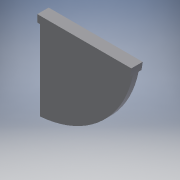
# Autodesk Inventor part: Control surface
Saved by Autodesk Inventor 2016 (Build 200138000, 138)
## iProperties
Created: 2015-09-03
Part Number: Control surface
Material: Generic
Document SubType Name: Modeling
Designer: Sudhar
Density: 1 g/cm^3
Appearance: Default
Author: Sudhar
Autodesk Inventor part; units mm, degrees
ref_plane "YZ Plane" through (0, 0, 0) normal (1, 0, 0) x (0, 1, 0)
ref_plane "XZ Plane" through (0, 0, 0) normal (0, 1, 0) x (-1, 0, 0)
ref_plane "XY Plane" through (0, 0, 0) normal (0, 0, 1) x (1, 0, 0)
sketch "Sketch1" plane through (0, 0, 0) normal (0, 0, 1) x (1, 0, 0)
  line L0 (12.2331, 11.5545) -> (-8.7602, 11.5545)
  line L1 (-8.7602, 11.5545) -> (-8.7602, -8.5579)
  arc A0 (-8.7602, -8.5579) -> (12.2331, 11.5545) centre (-10.663, 14.4408) ccw
  point P0 (0, 0)
  constraints: 4 end point, 2 point on circle, 1 centre point, 1 horizontal, 1 perpendicular
extrude "Extrusion1" add sketch "Sketch1" along normal mid plane 2.54
sketch "Sketch2" plane through (0, 0, 1.27) normal (0, 0, 1) x (1, 0, 0)
  line L0 (-8.7602, 11.5545) -> (-8.7602, -8.5579) projected
  line L1 (-8.7602, 9.9328) -> (11.9484, 9.8273)
  arc A0 (-8.7602, -8.5579) -> (12.2331, 11.5545) centre (-10.663, 14.4408) ccw projected
  point P0 (0, 0)
  constraints: 2 end point, 1 point on circle, 1 point on line
extrude "Extrusion2" cut sketch "Sketch2" against normal blind 0.635
sketch "Sketch3" plane through (0, 0, -1.27) normal (0, 0, -1) x (-1, 0, 0)
  line L0 (8.7602, 9.9328) -> (-11.9484, 9.8273) projected
  line L1 (8.7602, -8.5579) -> (8.7602, 11.5545) projected
  line L2 (8.7602, 9.9328) -> (8.7602, -8.5579)
  arc A0 (-11.9484, 9.8273) -> (8.7602, -8.5579) centre (10.663, 14.4408) ccw
  point P0 (0, 0)
  constraints: 2 end point, 2 point on circle, 1 centre point, 1 collinear
extrude "Extrusion3" cut sketch "Sketch3" against normal blind 0.635
body "Solid1"
